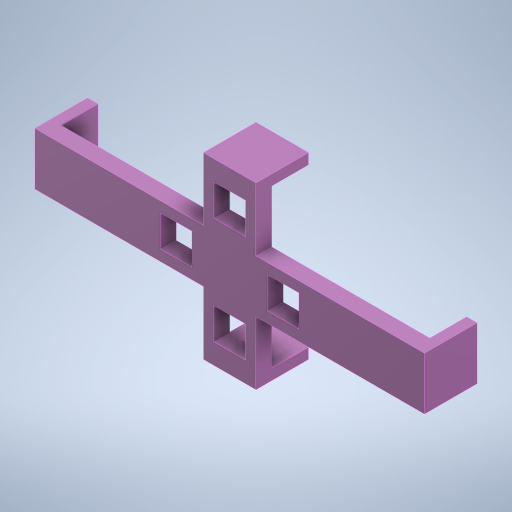
# Autodesk Inventor part: Центровщик кнопок
Saved by Autodesk Inventor 2024 (Build 280153020, 153B)
## iProperties
Created: 2023-06-11
Part Number: Центровщик кнопок
Material: Типовые
Document SubType Name: Modeling
Designer: Admin
Density: 1 g/cm^3
Appearance: По умолчанию
Author: Admin
Autodesk Inventor part; units mm, degrees
ref_plane "YZ Plane" through (0, 0, 0) normal (1, 0, 0) x (0, 1, 0)
ref_plane "XZ Plane" through (0, 0, 0) normal (0, 1, 0) x (-1, 0, 0)
ref_plane "XY Plane" through (0, 0, 0) normal (0, 0, 1) x (1, 0, 0)
sketch "Эскиз1" plane through (0, 0, 0) normal (0, 0, 1) x (1, 0, 0)
  line L0 (-3, 13.16) -> (3, 13.16)
  line L1 (3, 13.16) -> (3, 7.16)
  line L2 (3, 7.16) -> (-3, 7.16)
  line L3 (-3, 7.16) -> (-3, 13.16)
  line L4 (0, 0) -> (3.7075, 0) construction
  line L5 (-3, -13.16) -> (3, -13.16)
  line L6 (3, -13.16) -> (3, -7.16)
  line L7 (3, -7.16) -> (-3, -7.16)
  line L8 (-3, -7.16) -> (-3, -13.16)
  line L9 (-13.16, 3) -> (-7.16, 3)
  line L10 (-7.16, 3) -> (-7.16, -3)
  line L11 (-7.16, -3) -> (-13.16, -3)
  line L12 (-13.16, -3) -> (-13.16, 3)
  line L13 (0, 0) -> (0, 3.422) construction
  line L14 (7.16, -3) -> (13.16, -3)
  line L15 (13.16, -3) -> (13.16, 3)
  line L16 (13.16, 3) -> (7.16, 3)
  line L17 (7.16, 3) -> (7.16, -3)
  line L18 (-35, -5) -> (-5, -5)
  line L19 (-5, -5) -> (-5, -15)
  line L20 (5, -15) -> (5, -5)
  line L21 (5, -5) -> (35, -5)
  line L22 (35, 5) -> (5, 5)
  line L23 (5, 5) -> (5, 15)
  line L24 (-5, 15) -> (-5, 5)
  line L25 (-5, 5) -> (-35, 5)
  line L26 (-35, 15) -> (35, 15)
  line L27 (35, 15) -> (35, -15)
  line L28 (35, -15) -> (-35, -15)
  line L29 (-35, -15) -> (-35, 15)
  line L30 (-35, -5) -> (-37, -5)
  line L31 (-37, -5) -> (-37, 5)
  line L32 (-37, 5) -> (-35, 5)
  line L33 (-5, 15) -> (-5, 17)
  line L34 (-5, 17) -> (5, 17)
  line L35 (5, 17) -> (5, 15)
  line L36 (35, 5) -> (37, 5)
  line L37 (37, 5) -> (37, -5)
  line L38 (37, -5) -> (35, -5)
  line L39 (5, -15) -> (5, -17)
  line L40 (5, -17) -> (-5, -17)
  line L41 (-5, -17) -> (-5, -15)
  point P0 (3, 10.16)
  point P1 (0, 13.16)
  point P2 (3, -10.16)
  point P3 (0, -13.16)
  point P4 (-13.16, 0)
  point P5 (7.16, 0)
  point P6 (0, 7.16)
  point P7 (0, 15)
  point P8 (35, 0)
  point P9 (0, 10.16)
  point P10 (0, -10.16)
  point P11 (10.16, 0)
  point P12 (-10.16, 0)
  point P13 (3, -10.16)
  point P14 (10.16, 3)
  point P15 (-10.16, 3)
  dimension "Length" = 70
  dimension "Width" = 30
  dimension "d8" = 2
  dimension "d13" = 10.16
  dimension "d14" = 10.16
  dimension "d15" = 5
  dimension "d16" = 5
  constraints: 84 end point, 16 point on line, 12 perpendicular, 10 midpoint, 8 equal length, 8 horizontal alignment, 8 parallel, 6 horizontal, 6 symmetric about line, 6 vertical alignment, 3 vertical, 1 coincident, 1 collinear, 5 other
  measures "Length" distance of L26.start L26.end
  measures "Width" distance of L26.end L27.end
  measures "d8" distance of L18.start L30.end
  measures "d13" distance of point (0, 0) point (0, 10.16)
  measures "d14" distance of point (-10.16, 0) point (0, 0)
  measures "d15" distance from line of L23 point (0, 10.16)
  measures "d16" distance from line of L22 point (10.16, 0)
extrude "Выдавливание1" add sketch "Эскиз1" along normal blind 3 contours L29 L25 L24 L26 L23 L22 L27 L21 L20 L28 L19 L18 | L30 L31 L32 L29 | L28 L39 L40 L41 | L33 L34 L35 L26 | L27 L36 L37 L38
extrude "Выдавливание2" add sketch "Эскиз1" against normal blind 7 contours L30 L31 L32 L29 | L28 L39 L40 L41 | L33 L34 L35 L26 | L27 L36 L37 L38
